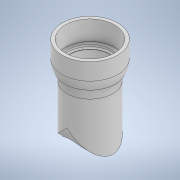
# Autodesk Inventor part: Modelo1_tronco_Pepu
Saved by Autodesk Inventor 2021 (Build 250183000, 183)
## iProperties
Created: 2020-12-04
Part Number: Modelo1_tronco_Pepu
Material: Genérico
Document SubType Name: Modeling
Designer: Joaquín
Density: 1 g/cm^3
Appearance: Valor por defecto
Author: Joaquín
Autodesk Inventor part; units mm, degrees
ref_plane "YZ Plane" through (0, 0, 0) normal (1, 0, 0) x (0, 1, 0)
ref_plane "XZ Plane" through (0, 0, 0) normal (0, 1, 0) x (-1, 0, 0)
ref_plane "XY Plane" through (0, 0, 0) normal (0, 0, 1) x (1, 0, 0)
sketch "Boceto1" plane through (0, 0, 0) normal (0, 1, 0) x (-1, 0, 0)
  circle A0 centre (0, 0) radius 30
  circle A1 centre (0, 0) radius 35
  dimension "d0" = 60
  dimension "d1" = 70
  constraints: 2 centre point, 2 coincident
  measures "d0" diameter of A0
  measures "d1" diameter of A1
extrude "Extrusión1" add sketch "Boceto1" along normal blind 100
sketch "Boceto2" plane through (0, 0, 0) normal (0, -1, 0) x (1, 0, 0)
  line L0 (0, 0) -> (0, 45)
  line L1 (45, 35) -> (45, -35)
  line L2 (40, 35) -> (40, -35)
  line L3 (45, 0) -> (45, -35)
  line L4 (45, -35) -> (40, -35)
  line L5 (45, 0) -> (45, 35)
  line L6 (45, 35) -> (40, 35)
  constraints: 14 end point, 2 perpendicular, 1 midpoint, 1 vertical
extrude "Extrusión2" add sketch "Boceto2" against normal blind 35
sketch "Boceto3" plane through (45, 0, 35) normal (1, 0, 0) x (0, 0, -1)
  line L0 (35, 0) -> (35, 35)
  circle A0 centre (35, 35) radius 35
  line L1 (0, 0) -> (0, 35) projected
  line L2 (0, 35) -> (0, 0)
  line L3 (70, 0) -> (0, 0) projected
  line L4 (0, 0) -> (70, 0)
  line L5 (70, 0) -> (70, 35) projected
  line L6 (70, 0) -> (70, 35)
  point P0 (70, 35)
  constraints: 8 end point, 2 perpendicular, 2 point on circle, 1 centre point, 1 coincident, 1 collinear, 1 tangent, 1 vertical
extrude "Extrusión3" cut sketch "Boceto3" against normal blind 100 contours L5 L3 A0 | A0 L3 L1
sketch "Boceto4" plane through (45, 35, 0) normal (1, 0, 0) x (0, 0, -1)
  line L0 (-35, 0) -> (35, 0) projected
  line L1 (-35, 0) -> (35, 0)
  point P0 (0, -35)
  constraints: 2 end point, 1 collinear
sketch "Boceto5" plane through (0, 35, 0) normal (0, 1, 0) x (1, 0, 0)
  line L0 (40, 35) -> (40, -35) projected
  line L1 (40, -35) -> (45, -35) projected
  line L2 (40, -35) -> (45, -35)
  line L3 (45, -35) -> (45, 35) projected
  line L4 (45, -35) -> (45, 35)
  line L5 (45, 35) -> (40, 35) projected
  line L6 (45, 35) -> (40, 35)
  line L7 (40, 35) -> (40, -35)
  point P0 (0, 0)
  constraints: 8 end point, 2 collinear, 2 perpendicular
extrude "Extrusión4" cut sketch "Boceto5" against normal blind 35
sketch "Boceto6" plane through (0, 100, 0) normal (0, 1, 0) x (1, 0, 0)
  circle A0 centre (0, 0) radius 42.5
  circle A1 centre (0, 0) radius 32.5
  dimension "d19" = 85
  dimension "d20" = 65
  constraints: 2 centre point, 2 coincident
  measures "d19" diameter of A0
  measures "d20" diameter of A1
extrude "Extrusión5" add sketch "Boceto6" along normal blind 35
fillet "Empalme1" radius 30 1 edges at (35, 100, 0)
fillet "Empalme2" radius 2 1 edges at (-32.5, 100, 0)
fillet "Empalme3" radius 30 2 edges at (0, 100, -42.5) (0, 100, 42.5)
sketch "Boceto7" plane through (0, 135, 0) normal (0, 1, 0) x (1, 0, 0)
  circle A0 centre (0, 0) radius 32.5
  circle A1 centre (0, 0) radius 37.5
  dimension "d26" = 75
  constraints: 2 centre point, 2 coincident
  measures "d26" diameter of A1
extrude "Extrusión6" cut sketch "Boceto7" against normal blind 30
